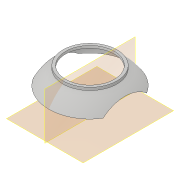
# Autodesk Inventor part: side
Saved by Autodesk Inventor 2017 (Build 210142000, 142)
## iProperties
Created: 2018-10-19
Part Number: side
Material: Generic
Document SubType Name: Modeling
Designer: jpb34
Density: 1 g/cm^3
Appearance: Default
Author: jpb34
Autodesk Inventor part; units mm, degrees
ref_plane "XY Plane" through (0, 0, 0) normal (0, 0, 1) x (1, 0, 0)
sketch "Sketch1" plane through (0, 0, 0) normal (0, 1, 0) x (-1, 0, 0)
  circle A0 centre (0, 0) radius 12.612
  line L0 (12.612, 0) -> (-12.612, 0)
  circle A1 centre (0, 0) radius 21.59
  dimension "d29" = 43.18
  constraints: 2 centre point, 2 coincident, 2 end point, 2 point on circle, 1 horizontal
  measures "d29" diameter of A1
revolve "Revolution1" add sketch "Sketch1" angle 360 about axis through (-12.612, 0, 0) along (1, 0, 0) contours L0 A0 | A0 L0
sketch "Sketch2" plane through (0, 0, 0) normal (0, 1, 0) x (-1, 0, 0)
  circle A0 centre (0, 0) radius 6.3549
  constraints: 1 centre point, 1 coincident
extrude "Extrusion1" cut sketch "Sketch2" along normal mid plane 25.4
hole "Hole1" [suppressed]
hole "Hole2" [suppressed]
sketch "Sketch3" plane through (0, 0, 0) normal (0, 1, 0) x (-1, 0, 0)
  point P0 (0, 0)
sketch "Sketch4" plane through (0, 0, 0) normal (1, 0, 0) x (0, 1, 0)
  line L0 (6.604, 13.4644) -> (-12.0538, 13.4644)
  line L1 (-12.0538, 13.4644) -> (-12.0538, -13.0797)
  line L2 (-12.0538, -13.0797) -> (6.604, -13.0797)
  line L3 (6.604, -13.0797) -> (6.604, 13.4644)
  point P0 (0, 0)
  constraints: 8 end point, 2 parallel, 1 horizontal, 1 perpendicular
extrude "Extrusion2" cut sketch "Sketch4" along normal mid plane 30.48
sketch "Sketch5" plane through (0, 0, 0) normal (1, 0, 0) x (0, 1, 0)
  circle A0 centre (0, 0) radius 8.7198
  constraints: 1 centre point, 1 coincident
extrude "Extrusion3" cut sketch "Sketch5" along normal mid plane 30.48
sketch "Sketch6" plane through (0, 0, 0) normal (0, 1, 0) x (-1, 0, 0)
  circle A0 centre (0, 0) radius 6.3549
  circle A1 centre (0, 0) radius 7.0528
  constraints: 2 centre point, 2 coincident
extrude "Extrusion4" add sketch "Sketch6" along normal blind 11.176
sketch "Sketch7" plane through (0, 0, 0) normal (0, 1, 0) x (-1, 0, 0)
  circle A0 centre (0, 0) radius 6.3549
  circle A1 centre (0, 0) radius 7.0528
  constraints: 2 centre point, 2 coincident
extrude "Extrusion5" cut sketch "Sketch7" along normal blind 10.16
sketch "Sketch8" plane through (0, 0, 0) normal (0, 1, 0) x (-1, 0, 0)
  point P0 (0, 0)
sketch "Sketch9" plane through (0, 0, 0) normal (0, 1, 0) x (-1, 0, 0)
  circle A0 centre (0, 0) radius 12.319
  line L0 (12.319, 0) -> (-12.319, 0)
  dimension "d30" = 24.638
  constraints: 2 end point, 2 point on circle, 1 centre point, 1 coincident, 1 horizontal
  measures "d30" diameter of A0
revolve "Revolution2" cut sketch "Sketch9" angle 360 about axis through (-12.319, 0, 0) along (1, 0, 0)
body "Solid1"
